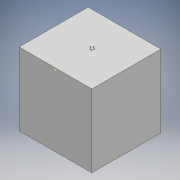
# Autodesk Inventor part: cubesat
Saved by Autodesk Inventor 2017 (Build 210142000, 142)
## iProperties
Created: 2016-12-14
Part Number: cubesat
Material: Generic
Document SubType Name: Modeling
Designer: Ali
Mass: 230.5 g
Surface Area: 942 cm^2
Volume: 230.5 cm^3
Density: 1 g/cm^3
Appearance: Default
Author: Ali
Autodesk Inventor part; units mm, degrees
ref_plane "YZ Plane" through (0, 0, 0) normal (1, 0, 0) x (0, 1, 0)
ref_plane "XZ Plane" through (0, 0, 0) normal (0, 1, 0) x (-1, 0, 0)
ref_plane "XY Plane" through (0, 0, 0) normal (0, 0, 1) x (1, 0, 0)
sketch "Sketch1" plane through (0, 0, 0) normal (0, 1, 0) x (-1, 0, 0)
  line L0 (50, -50) -> (-50, -50)
  line L1 (-50, -50) -> (-50, 50)
  line L2 (-50, 50) -> (50, 50)
  line L3 (50, 50) -> (50, -50)
  point P0 (0, 0)
  point P1 (0, 0)
  dimension "d0" = 100
  dimension "d1" = 100
  dimension "d2" = 50
  constraints: 8 end point, 2 parallel, 1 coincident, 1 horizontal, 1 perpendicular
  measures "d0" distance of L2.end L0.start
  measures "d1" distance of L0.start L0.end
  measures "d2" distance from line of L3 point (0, 0)
extrude "Extrusion1" add sketch "Sketch1" along normal blind 95
sketch "Sketch2" plane through (0, 95, 0) normal (0, 1, 0) x (1, 0, 0)
  line L0 (-45, 45) -> (45, 45)
  line L1 (45, 45) -> (45, -45)
  line L2 (45, -45) -> (-45, -45)
  line L3 (-45, -45) -> (-45, 45)
  line L4 (50, -50) -> (50, 50) projected
  line L5 (-50, 50) -> (-50, -50) projected
  line L6 (-50, -50) -> (50, -50) projected
  line L7 (-50, 50) -> (50, 50) projected
  point P0 (0, 0)
  dimension "d5" = 5
  dimension "d6" = 5
  dimension "d7" = 5
  dimension "d8" = 5
  constraints: 8 end point, 2 parallel, 1 horizontal, 1 perpendicular
  measures "d5" distance between parallel lines of L4 L1
  measures "d6" distance between parallel lines of L5 L3
  measures "d7" distance between parallel lines of L6 L2
  measures "d8" distance between parallel lines of L7 L0
extrude "Extrusion2" cut sketch "Sketch2" against normal blind 85 contours L0 L1 L2 L3
sketch "Sketch3" plane through (0, 95, 0) normal (0, 1, 0) x (1, 0, 0)
  line L0 (50, -50) -> (50, 50) projected
  circle A0 centre (47.5, 47.5) radius 1
  line L1 (-50, 50) -> (50, 50) projected
  line L2 (-50, -50) -> (50, -50) projected
  circle A1 centre (47.5, -47.5) radius 1
  line L3 (-50, 50) -> (-50, -50) projected
  circle A2 centre (-47.5, -47.5) radius 1
  circle A3 centre (-47.5, 47.5) radius 1
  point P0 (0, 0)
  point P1 (47.5, -47.5)
  dimension "d12" = 2.5
  dimension "d13" = 2.5
  dimension "d14" = 2.5
  dimension "d15" = 2.5
  dimension "d16" = 2
  dimension "d17" = 2.5
  dimension "d18" = 2.5
  dimension "d19" = 2.5
  dimension "d20" = 2.5
  constraints: 4 centre point, 4 coincident, 3 equal radius
  measures "d12" distance from line of L0 point (47.5, 47.5)
  measures "d13" distance from line of L1 point (47.5, 47.5)
  measures "d14" distance from line of L0 point (47.5, -47.5)
  measures "d15" distance from line of L2 point (47.5, -47.5)
  measures "d16" diameter of A0
  measures "d17" distance from line of L2 point (-47.5, -47.5)
  measures "d18" distance from line of L3 point (-47.5, -47.5)
  measures "d19" distance from line of L3 point (-47.5, 47.5)
  measures "d20" distance from line of L1 point (-47.5, 47.5)
hole "Hole2" at (47.5, 95, -47.5) at (47.5, 95, 47.5) at (-47.5, 95, 47.5) at (-47.5, 95, -47.5) direction (0, -1, 0) diameter 2 depth 8
sketch "Sketch9" plane through (-45, 95, 45) normal (1, 0, 0) x (0, 0, -1)
  circle A0 centre (45, -45) radius 10.5
  point P0 (45, -95)
  dimension "d66" = 21
  constraints: 1 centre point
  measures "d66" diameter of A0
extrude "Extrusion4" cut sketch "Sketch9" against normal blind 3
sketch "Sketch10" plane through (0, 10, 0) normal (0, 1, 0) x (1, 0, 0)
  circle A0 centre (0, 0) radius 10.5
  dimension "d69" = 21
  constraints: 1 centre point, 1 coincident
  measures "d69" diameter of A0
extrude "Extrusion5" cut sketch "Sketch10" against normal blind 3
sketch "Sketch11" plane through (45, 95, 45) normal (0, 0, -1) x (-1, 0, 0)
  circle A0 centre (45, -45) radius 10.5
  line L0 (0, 0) -> (0, -85) projected
  line L1 (0, 0) -> (90, 0) projected
  point P0 (45, -95)
  dimension "d72" = 45
  dimension "d73" = 45
  dimension "d74" = 21
  constraints: 1 centre point
  measures "d72" distance from line of L0 A0.centre
  measures "d73" distance from line of L1 A0.centre
  measures "d74" diameter of A0
extrude "Extrusion6" cut sketch "Sketch11" against normal blind 3
sketch "Sketch13" plane through (0, 50, 48) normal (0, 0, -1) x (-1, 0, 0)
  circle A0 centre (0, 0) radius 1.75
  point P0 (0, -50)
  dimension "d77" = 3.5
  constraints: 1 centre point
  measures "d77" diameter of A0
body "Solid1"
